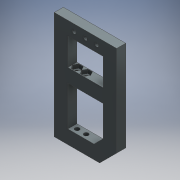
# Autodesk Inventor part: chassi_back_right
Saved by Autodesk Inventor 2016 (Build 200138000, 138)
## iProperties
Created: 2017-01-03
Part Number: chassi_back_right
Material: Generic
Document SubType Name: Modeling
Designer: hesaon
Density: 1 g/cm^3
Appearance: Default
Author: hesaon
Autodesk Inventor part; units mm, degrees
ref_plane "YZ Plane" through (0, 0, 0) normal (1, 0, 0) x (0, 1, 0)
ref_plane "XZ Plane" through (0, 0, 0) normal (0, 1, 0) x (-1, 0, 0)
ref_plane "XY Plane" through (0, 0, 0) normal (0, 0, 1) x (1, 0, 0)
sketch "Sketch1" plane through (0, 0, 0) normal (0, 1, 0) x (-1, 0, 0)
  line L0 (0, 142.5) -> (0, 0)
  line L1 (0, 142.5) -> (-82.5, 142.5)
  line L2 (0, 0) -> (-60, 0)
  line L3 (-60, 0) -> (-82.5, 22.5)
  line L4 (-82.5, 142.5) -> (-82.5, 22.5)
  line L5 (-18, 18) -> (-52.5442, 18)
  line L6 (-64.5, 124.5) -> (-18, 124.5)
  line L7 (-18, 88.5) -> (-64.5, 88.5)
  line L8 (-18, 70.5) -> (-64.5, 70.5)
  line L9 (-18, 124.5) -> (-18, 88.5)
  line L10 (-18, 70.5) -> (-18, 18)
  line L11 (-64.5, 29.9558) -> (-64.5, 70.5)
  line L12 (-64.5, 88.5) -> (-64.5, 124.5)
  line L13 (-52.5442, 18) -> (-64.5, 29.9558)
  dimension "d1" = 142.5
  dimension "d3" = 82.5
  dimension "d4" = 60
  dimension "d5" = 135
  dimension "d6" = 120
  dimension "d8" = 18
  dimension "d9" = 18
  dimension "d15" = 88.5
  dimension "d16" = 18
  dimension "d17" = 18
  dimension "d18" = 18
  dimension "d19" = 18
  dimension "d20" = 18
  dimension "d21" = 18
  constraints: 28 end point, 6 perpendicular, 3 vertical, 2 horizontal, 2 parallel, 1 coincident
  measures "d1" distance of L0.end L0.start
  measures "d3" distance of L0.start L1.end
  measures "d4" distance of L0.end L2.end
  measures "d5" angle of L2 L3
  measures "d6" distance of L3.end L1.end
  measures "d8" distance between parallel lines of L1 L6
  measures "d9" distance between parallel lines of L2 L5
  measures "d15" distance between parallel lines of L2 L7
  measures "d16" distance between parallel lines of L8 L7
  measures "d17" distance of L8.end L7.end
  measures "d18" distance from line of L0 L6.end
  measures "d19" distance between parallel lines of L0 L10
  measures "d20" distance between parallel lines of L4 L12
  measures "d21" distance between parallel lines of L3 L13
extrude "Extrusion2" add sketch "Sketch1" along normal blind 12
sketch "Sketch5" plane through (60, 0, 0) normal (0, 0, -1) x (-1, 0, 0)
  line L0 (42, 0) -> (42, 12) projected
  circle A0 centre (35.8, 6) radius 2.85
  circle A1 centre (23.8, 6) radius 2.85
  line L1 (0, 12) -> (60, 12) projected
  point P0 (60, 0)
  dimension "d35" = 5.7
  dimension "d36" = 5.7
  dimension "d37" = 6
  dimension "d38" = 6
  dimension "d39" = 6.2
  dimension "d40" = 12
  constraints: 2 centre point
  measures "d35" diameter of A0
  measures "d36" diameter of A1
  measures "d37" distance from line of L1 A0.centre
  measures "d38" distance from line of L1 A1.centre
  measures "d39" distance from line of L0 A0.centre
  measures "d40" distance of A0.centre A1.centre
extrude "Extrusion5" cut sketch "Sketch5" against normal up to surface (88.5 mm away) from surface at 0
sketch "Sketch6" plane through (18, 0, 88.5) normal (0, 0, 1) x (1, 0, 0)
  circle A0 centre (6.2, 6) radius 2.85 projected
  line L0 (9.2022, 11.2) -> (12.2044, 6)
  line L1 (12.2044, 6) -> (9.2022, 0.8)
  line L2 (9.2022, 0.8) -> (3.1978, 0.8)
  line L3 (3.1978, 0.8) -> (0.1956, 6)
  line L4 (0.1956, 6) -> (3.1978, 11.2)
  line L5 (3.1978, 11.2) -> (9.2022, 11.2)
  line L6 (21.2022, 11.2) -> (24.2044, 6)
  line L7 (24.2044, 6) -> (21.2022, 0.8)
  line L8 (21.2022, 0.8) -> (15.1978, 0.8)
  line L9 (15.1978, 0.8) -> (12.1956, 6)
  line L10 (12.1956, 6) -> (15.1978, 11.2)
  line L11 (15.1978, 11.2) -> (21.2022, 11.2)
  line L12 (46.5, 12) -> (0, 12) projected
  point P0 (-18, 0)
  point P1 (18.2, 6)
  point P2 (18.2, 11.2)
  dimension "d43" = 10.4
  dimension "d44" = 12
  constraints: 24 end point, 2 parallel, 1 coincident, 1 horizontal alignment, 1 midpoint, 1 point on line, 26 other
  measures "d43" distance between parallel lines of L5 L2
  measures "d44" distance of point (18.2, 6) point (6.2, 6)
extrude "Extrusion6" cut sketch "Sketch6" against normal blind 5
sketch "Sketch7" plane through (0, 0, 0) normal (0, -1, 0) x (1, 0, 0)
  circle A0 centre (26.25, 133.5) radius 2.5
  circle A1 centre (41.25, 133.5) radius 2.5
  circle A2 centre (56.25, 133.5) radius 2.5
  line L0 (18, 124.5) -> (64.5, 124.5) projected
  line L1 (18, 88.5) -> (18, 124.5) projected
  point P0 (0, 0)
  dimension "d47" = 5
  dimension "d48" = 5
  dimension "d49" = 5
  dimension "d50" = 15
  dimension "d51" = 15
  dimension "d52" = 9
  dimension "d53" = 8.25
  constraints: 3 centre point, 2 horizontal alignment
  measures "d47" diameter of A0
  measures "d48" diameter of A1
  measures "d49" diameter of A2
  measures "d50" distance of A1.centre A0.centre
  measures "d51" distance of A1.centre A2.centre
  measures "d52" distance from line of L0 A0.centre
  measures "d53" distance from line of A0.centre L1
extrude "Extrusion7" cut sketch "Sketch7" against normal up to next
body "Solid2"
